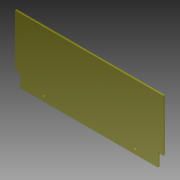
# Autodesk Inventor part: visor
Saved by Autodesk Inventor 2014 SP2 (Build 180246200, 246)
## iProperties
Created: 2016-05-05
Part Number: visor
Material: Generic
Document SubType Name: Modeling
Designer: cruiser
Density: 1 g/cm^3
Appearance: Clear - Yellow
Author: cruiser
Autodesk Inventor part; units mm, degrees
ref_plane "YZ Plane" through (0, 0, 0) normal (1, 0, 0) x (0, 1, 0)
ref_plane "XZ Plane" through (0, 0, 0) normal (0, 1, 0) x (-1, 0, 0)
ref_plane "XY Plane" through (0, 0, 0) normal (0, 0, 1) x (1, 0, 0)
sketch "Sketch1" plane through (0, 0, 0) normal (0, 1, 0) x (-1, 0, 0)
  line L0 (128.65, -55.5312) -> (-128.65, -55.5313)
  line L1 (-128.65, -55.5313) -> (-128.65, 55.5312)
  line L2 (-128.65, 55.5312) -> (128.65, 55.5313)
  line L3 (128.65, 55.5313) -> (128.65, -55.5312)
  line L4 (128.65, -55.5312) -> (-128.65, 55.5312) construction
  line L5 (-128.65, -55.5313) -> (128.65, 55.5313) construction
  point P0 (0, 0)
  dimension "d0" = 257.3
  dimension "d1" = 111.0625
  constraints: 12 end point, 2 midpoint, 2 parallel, 1 horizontal, 1 perpendicular
  measures "d0" distance of L1.end L2.end
  measures "d1" distance of L0.end L1.end
extrude "Extrusion1" add sketch "Sketch1" along normal blind 3.15
sketch "Sketch3" plane through (0, 0, 0) normal (0, -1, 0) x (1, 0, 0)
  line L0 (-128.65, -55.5312) -> (128.65, -55.5313) projected
  line L1 (128.65, -55.5313) -> (128.65, 55.5312) projected
  line L2 (128.65, 55.5312) -> (-128.65, 55.5313) projected
  line L3 (-128.65, 55.5313) -> (-128.65, -55.5312) projected
  line L4 (138.65, -31.5312) -> (-138.65, -31.5313)
  line L5 (-138.65, -31.5313) -> (-138.65, 65.5312)
  line L6 (-138.65, 65.5312) -> (138.65, 65.5313)
  line L7 (138.65, 65.5313) -> (138.65, -31.5312)
  line L8 (138.65, -31.5312) -> (-138.65, 65.5312) construction
  line L9 (-138.65, -31.5313) -> (138.65, 65.5313) construction
  line L10 (113.7471, -115.5313) -> (-113.7471, -115.5313)
  line L11 (-113.7471, -115.5313) -> (-113.7471, -35.5313)
  line L12 (-113.7471, -35.5313) -> (113.7471, -35.5312)
  line L13 (113.7471, -35.5312) -> (113.7471, -115.5313)
  line L14 (113.7471, -115.5313) -> (-113.7471, -35.5313) construction
  line L15 (-113.7471, -115.5313) -> (113.7471, -35.5312) construction
  line L16 (160.8369, -119.5313) -> (-160.8369, -119.5313)
  line L17 (-160.8369, -119.5313) -> (-160.8369, -31.5313)
  line L18 (-160.8369, -31.5313) -> (160.8369, -31.5312)
  line L19 (160.8369, -31.5312) -> (160.8369, -119.5313)
  line L20 (160.8369, -119.5313) -> (-160.8369, -31.5313) construction
  line L21 (-160.8369, -119.5313) -> (160.8369, -31.5312) construction
  line L22 (0, 55.5313) -> (0, -55.5313)
  point P0 (0, 0)
  point P1 (0, 17)
  point P2 (0, -75.5313)
  dimension "d9" = 10
  dimension "d10" = 10
  dimension "d11" = 10
  dimension "d15" = 20
  dimension "d16" = 88
  dimension "d17" = 80
  dimension "d18" = 0
  dimension "d19" = 0
  constraints: 38 end point, 8 midpoint, 6 parallel, 3 horizontal, 3 perpendicular
  measures "d9" distance between parallel lines of L3 L5
  measures "d10" distance between parallel lines of L7 L1
  measures "d11" distance between parallel lines of L6 L2
  measures "d15" distance between parallel lines of L12 L0
  measures "d16" distance of L16.end L17.end
  measures "d17" distance of L10.end L11.end
  measures "d18" distance from line of L22 point (0, -75.531)
  measures "d19" distance between parallel lines of L18 L4
extrude "Extrusion3" add sketch "Sketch3" against normal blind 3.15 contours L4 L5 L6 L7 L1 L2 L3 | L3 L2 L22 L4 | L22 L2 L1 L4
sketch "Sketch2" plane through (0, 3.15, 0) normal (0, 1, 0) x (1, 0, 0)
  line L0 (128.65, 55.5313) -> (-128.65, 55.5312) projected
  circle A0 centre (-85.7667, 45.5313) radius 2.5
  line L1 (0, 0) -> (0, 55.5313)
  circle A1 centre (85.7667, 45.5313) radius 2.5
  dimension "d4" = 5
  dimension "d5" = 10
  dimension "d6" = 85.7667
  constraints: 2 centre point, 2 end point, 1 midpoint, 1 symmetric about line, 1 other
  measures "d4" diameter of A0
  measures "d5" distance from line of L0 A0.centre
  measures "d6" distance from line of L1 A0.centre
extrude "Extrusion2" cut sketch "Sketch2" against normal blind 3.15
equation "\"d0\" = visor_x"
equation "\"d1\" = visor_y"
equation "\"d2\" = clear_acrylic"
equation "\"d9\" = protection_slot_width"
equation "\"d10\" = protection_slot_width"
equation "\"d11\" = protection_slot_width"
equation "\"d15\" = visor_overlap"
equation "\"d16\" = 2 * frame_face_y"
equation "\"d17\" = frame_y"
equation "\"d13\" = clear_acrylic"
equation "\"d4\" = m5_diameter"
equation "\"d5\" = 0.5 * visor_overlap"
equation "\"d6\" = 0.333333 * visor_x"
equation "\"d7\" = clear_acrylic"
equation "\"sm_thickness\" = 1.5875"
equation "\"very_thick_acrylic\" = 9.45"
equation "\"thick_acrylic\" = 5.88"
equation "\"thin_acrylic\" = 3.15"
equation "\"clear_acrylic\" = 3.15"
equation "\"wood_thickness\" = 6.72"
equation "\"m3_diameter\" = 3"
equation "\"m4_diameter\" = 4"
equation "\"m5_diameter\" = 5"
equation "\"brass_insert_drill\" = 4"
equation "\"m5_brass_insert_drill\" = 6.7"
equation "\"m3_main_length\" = 14"
equation "\"m3_main_nut_width\" = 5.7"
equation "\"m3_main_nut_thickness\" = 2.5"
equation "\"m3_main_extra\" = 1"
equation "\"stepper_screw_space\" = 35"
equation "\"stepper_shaft_diameter\" = 5"
equation "\"stepper_body_diameter\" = 28"
equation "\"laser_body_diameter\" = 12"
equation "\"t_carrier\" = 5.88"
equation "\"t_wall\" = 5.88"
equation "\"t_window\" = 3.15"
equation "\"carrier_y\" = 251"
equation "\"carrier_z\" = 12"
equation "\"carrier_z2\" = 328.24"
equation "\"protection_slot\" = 44.2"
equation "\"protection_slot_offset\" = 55.25"
equation "\"window_z\" = 333.9125"
equation "\"window_y\" = 92.0625"
equation "\"door_sensor\" = 35"
equation "\"reservoir_x\" = 201"
equation "\"reservoir_y\" = 201"
equation "\"linear_bearing_spacing\" = 271"
equation "\"motor_spacing\" = 337"
equation "\"t_tray\" = 3.15"
equation "\"tray_border\" = 25"
equation "\"tray_x\" = 251"
equation "\"tray_y\" = 251"
equation "\"bed_z\" = 25"
equation "\"brass_keep_out\" = 8"
equation "\"tape_keep_out\" = 2"
equation "\"tape_thickness\" = 2"
equation "\"t_crane\" = 6.72"
equation "\"crane_z2\" = 12"
equation "\"end_stop_spacing\" = 19"
equation "\"thumb_nut_offset_y\" = 0"
equation "\"thumb_nut_diameter\" = 7"
equation "\"z_min_from_center\" = 115"
equation "\"t_frame\" = 6.72"
equation "\"frame_top_z\" = 385"
equation "\"frame_bottom_z\" = 275"
equation "\"frame_total_z\" = 661.5875"
equation "\"frame_y\" = 80"
equation "\"frame_border\" = 46.35"
equation "\"frame_foot_z\" = 12"
equation "\"frame_tilt\" = 1deg"
equation "\"printer_z\" = 289"
equation "\"lcd_x\" = 72"
equation "\"lcd_y\" = 25"
equation "\"subframe_x\" = 343"
equation "\"subframe_y_offset\" = 27.5"
equation "\"laser_y_offset\" = 19.4"
equation "\"laser_diameter\" = 12"
equation "\"laser_z_offset\" = 55"
equation "\"laser_y\" = 15"
equation "\"laser_z\" = 75"
equation "\"t_galvo_frame\" = 6.72"
equation "\"galvo_frame_x\" = 66"
equation "\"galvo_frame_z\" = 65"
equation "\"galvo_frame_y_offset\" = 27.5"
equation "\"drawer_x\" = 257.3"
equation "\"drawer_y\" = 88.65"
equation "\"drawer_z\" = 278.175"
equation "\"drawer_z_from_bottom\" = 25"
equation "\"nema17_x\" = 43"
equation "\"visor_y\" = 111.0625"
equation "\"visor_overlap\" = 20"
equation "\"visor_x\" = 257.3"
equation "\"door_z\" = 333.9125"
equation "\"door_x\" = 251"
equation "\"window_overlap\" = 48"
equation "\"door_overlap\" = 48"
equation "\"acrylic_into_frame\" = 5"
equation "\"protection_slot_width\" = 10"
equation "\"m3_press_nut_drill\" = 4.5"
equation "\"m3_head\" = 6"
equation "\"m5_press_nut_drill\" = 6.5"
equation "\"drawer_support_from_top\" = 48"
equation "\"laser_gap\" = 1"
equation "\"frame_screw_from_center\" = 25"
equation "\"drawer_screw_from_center\" = 54"
equation "\"drawer_screw_z\" = 145"
equation "\"frame_face_y\" = 44"
equation "\"switch_spacing\" = 19"
equation "\"subframe_y\" = 55"
body "Solid1"
